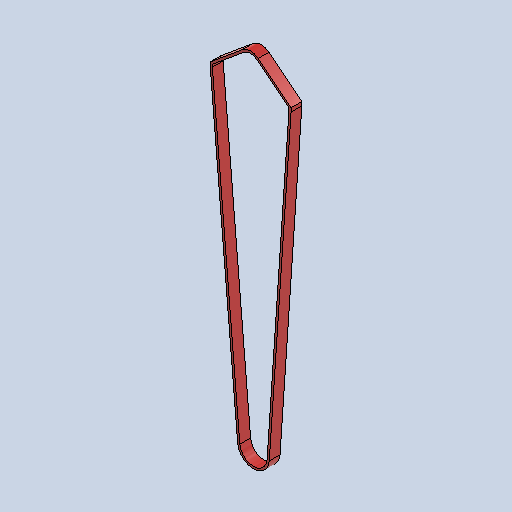
# Autodesk Inventor part: Compression bar band
Saved by Autodesk Inventor 2023.2 (Build 272271030, 271C)
## iProperties
Created: 2023-04-07
Part Number: Compression bar band
Material: Generic
Document SubType Name: Modeling
Designer: Main Account
Density: 1 g/cm^3
Appearance: Default
Author: Main Account
Autodesk Inventor part; units mm, degrees
ref_plane "YZ Plane" through (0, 0, 0) normal (1, 0, 0) x (0, 1, 0)
ref_plane "XZ Plane" through (0, 0, 0) normal (0, 1, 0) x (-1, 0, 0)
ref_plane "XY Plane" through (0, 0, 0) normal (0, 0, 1) x (1, 0, 0)
sketch "Sketch1" plane through (0, 0, 0) normal (0, 0, 1) x (1, 0, 0)
  circle A0 centre (-6, 6) radius 6.35 construction
  arc A1 (-12.3256, 5.444) -> (0.3346, 5.558) centre (-6, 6) ccw
  circle A2 centre (-7.3895, 160.2669) radius 4.7625 construction
  arc A3 (-4.4126, 163.9844) -> (-10.4328, 163.9301) centre (-7.3895, 160.2669) ccw
  line L0 (-25.083, 150.5821) -> (-25.0935, 151.7505) construction
  line L1 (10.465, 152.0707) -> (10.4756, 150.9024) construction
  line L2 (-10.4328, 163.9301) -> (-25.0935, 151.7505)
  line L3 (0.3346, 5.558) -> (10.4756, 150.9024)
  line L4 (10.465, 152.0707) -> (10.4756, 150.9024)
  line L5 (10.465, 152.0707) -> (-4.4126, 163.9844)
  line L6 (-25.0935, 151.7505) -> (-25.083, 150.5821)
  line L7 (-25.083, 150.5821) -> (-12.3256, 5.444)
  line L8 (11.4759, 150.8721) -> (1.3322, 5.4884)
  arc A4 (-13.3218, 5.3564) -> (1.3322, 5.4884) centre (-6, 6) ccw
  line L9 (-13.3218, 5.3564) -> (-26.0826, 150.5338)
  line L10 (-26.0826, 150.5338) -> (-26.0977, 152.2162)
  line L11 (-26.0977, 152.2162) -> (-11.0719, 164.6993)
  arc A5 (-3.7876, 164.7649) -> (-11.0719, 164.6993) centre (-7.3895, 160.2669) ccw
  line L12 (-3.7876, 164.7649) -> (11.4607, 152.5545)
  line L13 (11.4607, 152.5545) -> (11.4759, 150.8721)
  point P0 (0, 0)
  dimension "d7" = 1
  constraints: 24 end point, 8 point on circle, 4 centre point, 4 tangent, 2 coincident, 2 concentric, 1 collinear, 7 other
  measures "d7" distance between parallel lines of L3 L8
extrude "Extrusion1" add sketch "Sketch1" along normal blind 5
body "Solid1"
